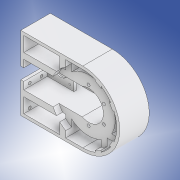
# Autodesk Inventor part: SJ001
Saved by Autodesk Inventor 2017 SP1 (Build 210196100, 196)
## iProperties
Created: 2017-06-03
Part Number: SJ001
Material: ABS Plastic
Document SubType Name: Modeling
Designer: Zach
Density: 1.06 g/cm^3
Appearance: CR White
Author: Zach
Autodesk Inventor part; units mm, degrees
ref_plane "YZ Plane" through (0, 0, 0) normal (1, 0, 0) x (0, 1, 0)
ref_plane "XZ Plane" through (0, 0, 0) normal (0, 1, 0) x (-1, 0, 0)
ref_plane "XY Plane" through (0, 0, 0) normal (0, 0, 1) x (1, 0, 0)
sketch "Sketch1" plane through (0, 0, 0) normal (0, 0, 1) x (1, 0, 0)
  circle A0 centre (0, 0) radius 62.5 construction
  line L0 (0, 62.5) -> (-105, 62.5)
  line L1 (-105, 62.5) -> (-105, -62.5)
  line L2 (-105, -62.5) -> (0, -62.5)
  arc A1 (0, -62.5) -> (0, 62.5) centre (0, 0) ccw
  dimension "d0" = 125
  dimension "d1" = 105
  constraints: 6 end point, 4 point on circle, 4 tangent, 2 centre point, 2 vertical alignment, 1 coincident, 1 concentric, 1 horizontal, 1 perpendicular
  measures "d0" diameter of A0
  measures "d1" distance of L0.start L0.end
extrude "Extrusion1" add sketch "Sketch1" along normal blind 50
sketch "Sketch6" plane through (0, 0, 50) normal (0, 0, 1) x (1, 0, 0)
  circle A0 centre (0, 0) radius 22.5
  arc A1 (0, -62.5) -> (0, 62.5) centre (0, 0) ccw projected
  dimension "d125" = 45
  constraints: 1 centre point, 1 coincident
  measures "d125" diameter of A0
extrude "Extrusion6" cut sketch "Sketch6" against normal blind 40
sketch "Sketch7" plane through (0, 0, 50) normal (0, 0, 1) x (1, 0, 0)
  line L0 (0, 10) -> (-105, 10)
  line L1 (-105, 10) -> (-105, -10)
  line L2 (-105, -10) -> (0, -10)
  line L3 (0, -10) -> (0, 10)
  circle A0 centre (0, 0) radius 22.5 projected
  line L4 (-105, 62.5) -> (-105, -62.5) projected
  point P0 (-105, 0)
  dimension "d28" = 20
  constraints: 8 end point, 3 midpoint, 2 parallel, 1 coincident, 1 horizontal, 1 perpendicular
  measures "d28" distance of L1.end L0.end
extrude "Extrusion7" cut sketch "Sketch7" against normal blind 40 contours L3 L2 A0 L0 | A0 L2 L1 L0 picked at (-7.5, 0)
sketch "Sketch9" plane through (0, 0, 50) normal (0, 0, 1) x (1, 0, 0)
  circle A0 centre (0, 30) radius 2.5
  circle A1 centre (-25.9808, 15) radius 2.5
  circle A2 centre (-25.9808, -15) radius 2.5
  circle A3 centre (0, -30) radius 2.5
  circle A4 centre (25.9808, -15) radius 2.5
  circle A5 centre (25.9808, 15) radius 2.5
  circle A6 centre (0, 0) radius 30 construction
  dimension "d123" = 60
  dimension "d35" = 5
  dimension "d39" = 360
  constraints: 6 centre point, 2 vertical alignment, 1 coincident, 15 other
  measures "d35" diameter of A0
extrude "Extrusion9" cut sketch "Sketch9" against normal through all
sketch "Sketch10" plane through (0, 0, 50) normal (0, 0, 1) x (1, 0, 0)
  circle A0 centre (0, 0) radius 45
  arc A1 (0, -57.5) -> (0, -57.5) centre (0, 0) ccw
  line L0 (0, -57.5) -> (-100, -57.5)
  line L1 (-100, 57.5) -> (-100, -57.5)
  line L2 (0, -57.5) -> (-75, -57.5)
  line L3 (0, 57.5) -> (-100, 57.5)
  circle A2 centre (0, 0) radius 57.5 construction
  arc A3 (0, -57.5) -> (0, 57.5) centre (0, 0) ccw
  line L4 (0, 62.5) -> (-105, 62.5) construction
  line L5 (-105, 62.5) -> (-105, 10) construction
  line L6 (-105, -10) -> (-105, 10) construction
  line L7 (-105, -10) -> (-105, -62.5) construction
  line L8 (-105, -62.5) -> (0, -62.5) construction
  arc A4 (0, -62.5) -> (0, 62.5) centre (0, 0) ccw construction
  point P0 (-100, 0)
  dimension "d111" = 115
  dimension "d43" = 90
  dimension "d114" = 90
  dimension "d124" = 5
  dimension "d212" = 5
  dimension "d213" = 5
  constraints: 8 end point, 4 point on circle, 3 centre point, 3 coincident, 2 tangent, 1 midpoint, 1 perpendicular, 1 vertical alignment, 3 other
  measures "d43" diameter of A0
  measures "d114" angle of L1 L3
  measures "d124" distance between parallel lines of L4 L3
  measures "d212" distance between parallel lines of L8 L0
  measures "d213" distance from line of L6 point (-100, 0)
extrude "Extrusion10" cut sketch "Sketch10" against normal blind 40
sketch "Sketch18" plane through (-105, -62.5, 0) normal (-1, 0, 0) x (0, 0, 1)
  circle A0 centre (40, 45) radius 2.5
  circle A1 centre (20, 45) radius 2.5
  line L0 (0, 125) -> (0, 0)
  circle A2 centre (40, 80) radius 2.5
  circle A3 centre (20, 80) radius 2.5
  circle A4 centre (20, 116.25) radius 2.5
  circle A5 centre (20, 8.75) radius 2.5
  circle A6 centre (40, 8.75) radius 2.5
  circle A7 centre (40, 116.25) radius 2.5
  line L1 (0, 125) -> (50, 125)
  line L2 (10, 87.5) -> (50, 87.5)
  line L3 (10, 52.5) -> (50, 52.5)
  line L4 (0, 0) -> (50, 0)
  line L5 (50, 52.5) -> (50, 37.5)
  point P0 (0, 62.5)
  dimension "d76" = 5
  dimension "d77" = 5
  dimension "d80" = 20
  dimension "d91" = 5
  dimension "d92" = 5
  dimension "d94" = 5
  dimension "d95" = 5
  dimension "d96" = 5
  dimension "d97" = 5
  dimension "d115" = 8.75
  dimension "d116" = 7.5
  dimension "d118" = 8.75
  dimension "d129" = 7.5
  constraints: 12 end point, 8 centre point, 6 vertical alignment, 4 horizontal alignment
  measures "d76" diameter of A0
  measures "d77" diameter of A1
  measures "d80" distance of A1.centre A0.centre
  measures "d91" diameter of A2
  measures "d92" diameter of A3
  measures "d94" diameter of A4
  measures "d95" diameter of A5
  measures "d96" diameter of A6
  measures "d97" diameter of A7
  measures "d115" distance from line of L1 A7.centre
  measures "d116" distance from line of L2 A2.centre
  measures "d118" distance from line of L4 A6.centre
  measures "d129" distance from line of A0.centre L3
extrude "Extrusion39" cut sketch "Sketch18" against normal blind 10
sketch "Sketch46" plane through (0, 0, 10) normal (0, 0, 1) x (1, 0, 0)
  arc A0 (-43.8748, -10) -> (-43.8748, 10) centre (0, 0) ccw construction
  line L0 (-45, 22.5) -> (-100, 22.5)
  line L1 (-31.1247, 32.5) -> (-100, 32.5)
  line L2 (-100, 32.5) -> (-100, 22.5)
  line L3 (-100, 22.5) -> (-31.1247, 22.5)
  line L4 (-31.1247, 22.5) -> (-31.1247, 32.5)
  line L5 (-135.4871, 0) -> (135.4871, 0) construction
  line L6 (-95, 57.5) -> (0, 57.5) construction
  line L7 (-38.9711, 22.5) -> (-28.9711, 22.5)
  line L8 (-28.9711, 22.5) -> (-28.9711, 57.5)
  line L9 (-28.9711, 57.5) -> (-38.9711, 57.5)
  line L10 (-38.9711, 57.5) -> (-38.9711, 22.5)
  arc A1 (0, -57.5) -> (0, 57.5) centre (0, 0) ccw construction
  line L11 (31.1247, 32.5) -> (52.915, 32.5)
  line L12 (52.915, 32.5) -> (52.915, 22.5)
  line L13 (52.915, 22.5) -> (31.1247, 22.5)
  line L14 (31.1247, 22.5) -> (31.1247, 32.5)
  line L15 (31.1247, 22.5) -> (21.1247, 22.5)
  line L16 (21.1247, 22.5) -> (21.1247, 53.4789)
  line L17 (21.1247, 53.4789) -> (31.1247, 53.4789)
  line L18 (31.1247, 53.4789) -> (31.1247, 22.5)
  line L19 (-45, -22.5) -> (-100, -22.5)
  line L20 (-31.1247, -32.5) -> (-100, -32.5)
  line L21 (-100, -32.5) -> (-100, -22.5)
  line L22 (-100, -22.5) -> (-31.1247, -22.5)
  line L23 (-31.1247, -22.5) -> (-31.1247, -32.5)
  line L24 (-28.9711, -22.5) -> (-28.9711, -57.5)
  line L25 (-28.9711, -57.5) -> (-38.9711, -57.5)
  line L26 (-38.9711, -57.5) -> (-38.9711, -22.5)
  line L27 (31.1247, -32.5) -> (52.915, -32.5)
  line L28 (52.915, -32.5) -> (52.915, -22.5)
  line L29 (52.915, -22.5) -> (31.1247, -22.5)
  line L30 (31.1247, -22.5) -> (31.1247, -32.5)
  line L31 (31.1247, -22.5) -> (21.1247, -22.5)
  line L32 (21.1247, -22.5) -> (21.1247, -53.4789)
  line L33 (21.1247, -53.4789) -> (31.1247, -53.4789)
  line L34 (31.1247, -53.4789) -> (31.1247, -22.5)
  line L35 (-28.9711, -22.5) -> (-38.9711, -22.5)
  line L36 (-100, -22.5) -> (5, -22.5) construction
  line L37 (-100, 10) -> (-100, 57.5) construction
  arc A2 (-43.8748, -10) -> (-43.8748, 10) centre (0, 0) ccw projected
  dimension "d229" = 10
  dimension "d230" = 10
  dimension "d231" = 10
  dimension "d232" = 10
  constraints: 74 end point, 15 symmetric about line, 11 point on circle, 8 parallel, 5 horizontal, 4 perpendicular, 3 point on line, 2 centre point, 1 coincident, 1 collinear, 1 horizontal alignment, 1 midpoint
  measures "d229" distance of L1.end L0.end
  measures "d230" distance of L9.end L8.end
  measures "d231" distance of L11.end L12.end
  measures "d232" distance of L16.end L17.end
extrude "Extrusion44" add sketch "Sketch46" along normal blind 40
sketch "Sketch22" plane through (0, 0, 50) normal (0, 0, 1) x (1, 0, 0)
  arc A0 (0, -62.5) -> (0, 62.5) centre (0, 0) ccw projected
  circle A1 centre (0, 0) radius 55
  point P0 (0, 0)
  dimension "d122" = 110
  constraints: 1 centre point, 1 coincident
  measures "d122" diameter of A1
extrude "Extrusion20" cut sketch "Sketch22" against normal blind 10
sketch "Sketch30" plane through (0, 0, 0) normal (0, 0, -1) x (-1, 0, 0)
  circle A0 centre (0, 0) radius 42.5 construction
  line L0 (0, 42.5) -> (105, 42.5)
  line L1 (105, 62.5) -> (105, -62.5) projected
  line L2 (0, -42.5) -> (105, -42.5)
  line L3 (105, 42.5) -> (105, -42.5)
  arc A1 (0, 42.5) -> (0, -42.5) centre (0, 0) ccw
  line L4 (100, 22.5) -> (0, 22.5)
  arc A2 (0, 22.5) -> (0, -22.5) centre (0, 0) ccw
  line L5 (0, -22.5) -> (100, -22.5)
  line L6 (100, -22.5) -> (100, 22.5)
  dimension "d162" = 85
  dimension "d201" = 45
  dimension "d202" = 5
  constraints: 12 end point, 6 point on circle, 3 centre point, 2 parallel, 2 point on line, 2 tangent, 1 coincident, 1 collinear, 1 concentric, 1 horizontal, 2 other
  measures "d162" diameter of A0
  measures "d201" distance between parallel lines of L5 L4
  measures "d202" distance between parallel lines of L1 L6
extrude "Extrusion29" add sketch "Sketch30" along normal blind 5
sketch "Sketch32" plane through (0, 0, 0) normal (0, 0, -1) x (-1, 0, 0)
  arc A0 (0, 22.5) -> (0, -22.5) centre (0, 0) ccw projected
  circle A1 centre (0, 0) radius 22.5 construction
  line L0 (0, 22.5) -> (100, 22.5)
  line L1 (100, -22.5) -> (100, 22.5) projected
  line L2 (0, -22.5) -> (100, -22.5)
  line L3 (100, 22.5) -> (100, -22.5)
  arc A2 (0, 22.5) -> (0, -22.5) centre (0, 0) ccw
  point P0 (0, 0)
  dimension "d168" = 45
  constraints: 6 end point, 4 point on circle, 3 tangent, 2 centre point, 2 horizontal, 2 point on line, 1 coincident, 1 collinear
  measures "d168" diameter of A1
extrude "Extrusion30" cut sketch "Sketch32" against normal through all
sketch "Sketch33" plane through (0, 0, -5) normal (0, 0, -1) x (-1, 0, 0)
  line L0 (100, 22.5) -> (100, -22.5) projected
  line L1 (100, -22.5) -> (0, -22.5) projected
  arc A0 (0, 22.5) -> (0, -22.5) centre (0, 0) ccw projected
  line L2 (0, 22.5) -> (100, 22.5) projected
  arc A1 (0, 42.5) -> (0, -42.5) centre (0, 0) ccw projected
  line L3 (0, -42.5) -> (105, -42.5) projected
  line L4 (105, -42.5) -> (105, 42.5) projected
  line L5 (105, 42.5) -> (0, 42.5) projected
  point P0 (0, 0)
extrude "Extrusion31" add sketch "Sketch33" along normal blind 5 contours L0 L1 A0 L2 | L5 L4 L3 A1
sketch "Sketch37" plane through (0, 0, 10) normal (0, 0, 1) x (1, 0, 0)
  circle A0 centre (0, 0) radius 15
  circle A1 centre (-77.5, 0) radius 12.5
  line L0 (-100, 22.5) -> (-100, -22.5)
  line L1 (-100, -22.5) -> (5, -22.5)
  arc A2 (5, -22.5) -> (5, 22.5) centre (5, 0) ccw
  line L2 (5, 22.5) -> (-100, 22.5)
  line L3 (-93, -15.5) -> (-62, -15.5) construction
  line L4 (-62, -15.5) -> (-62, 15.5) construction
  line L5 (-62, 15.5) -> (-93, 15.5) construction
  line L6 (-93, 15.5) -> (-93, -15.5) construction
  circle A3 centre (-77.5, 0) radius 3 construction
  line L7 (-93, -15.5) -> (-62, 15.5) construction
  line L8 (-62, -15.5) -> (-93, 15.5) construction
  line L9 (-100, -22.5) -> (-55, -22.5)
  line L10 (-55, -22.5) -> (-55, 22.5)
  line L11 (-55, 22.5) -> (-100, 22.5)
  line L12 (-100, 22.5) -> (-100, -22.5)
  line L13 (-100, -22.5) -> (-55, 22.5) construction
  line L14 (-55, -22.5) -> (-100, 22.5) construction
  circle A4 centre (-77.5, 0) radius 3
  circle A5 centre (-62, 15.5) radius 1.5
  circle A6 centre (-93, 15.5) radius 1.5
  circle A7 centre (-93, -15.5) radius 1.5
  circle A8 centre (-62, -15.5) radius 1.5
  point P0 (-77.5, 0)
  dimension "d188" = 31
  dimension "d189" = 45
  dimension "d191" = 31
  dimension "d192" = 6
  dimension "d193" = 3
  dimension "d194" = 3
  dimension "d195" = 3
  dimension "d196" = 3
  dimension "d242" = 25
  constraints: 30 end point, 9 centre point, 8 midpoint, 7 coincident, 4 parallel, 2 horizontal, 2 perpendicular, 2 point on circle
  measures "d188" distance of L5.end L4.end
  measures "d189" distance of L0.start L10.end
  measures "d191" distance of L3.end L4.end
  measures "d192" diameter of A4
  measures "d193" diameter of A5
  measures "d194" diameter of A6
  measures "d195" diameter of A7
  measures "d196" diameter of A8
  measures "d242" diameter of A1
extrude "Extrusion35" add sketch "Sketch37" against normal blind 5 contours L2 L10 L1 L0
sketch "Sketch39" plane through (0, 0, -10) normal (0, 0, -1) x (-1, 0, 0)
  circle A0 centre (77.5, 0) radius 3
  circle A1 centre (77.5, 0) radius 12.5 projected
  circle A2 centre (62, -15.5) radius 1.5 projected
  circle A3 centre (93, -15.5) radius 1.5 projected
  circle A4 centre (93, 15.5) radius 1.5 projected
  circle A5 centre (62, 15.5) radius 1.5 projected
  line L0 (55, -22.5) -> (55, 22.5) construction
  line L1 (100, 22.5) -> (55, 22.5) construction
  circle A6 centre (62, -15.5) radius 1.5 projected
  circle A7 centre (93, -15.5) radius 1.5 projected
  circle A8 centre (93, 15.5) radius 1.5 projected
  circle A9 centre (40.5, 0) radius 4
  circle A10 centre (0, 0) radius 22.5 construction
  circle A11 centre (40.5, 0) radius 22.5 construction
  line L2 (55, -22.5) -> (100, -22.5) projected
  line L3 (105, 10) -> (100, 10) projected
  line L4 (105, -10) -> (105, 10) projected
  line L5 (100, -10) -> (105, -10) projected
  line L6 (100, -22.5) -> (100, -10) projected
  line L7 (100, 10) -> (100, 22.5) projected
  circle A12 centre (0, 0) radius 4
  dimension "d217" = 6
  dimension "d218" = 37
  dimension "d219" = 8
  dimension "d222" = 45
  dimension "d223" = 45
  dimension "d235" = 8
  constraints: 5 centre point, 4 coincident, 1 horizontal alignment
  measures "d217" diameter of A0
  measures "d218" distance of A0.centre A9.centre
  measures "d219" diameter of A9
  measures "d222" diameter of A10
  measures "d223" diameter of A11
  measures "d235" diameter of A12
extrude "Extrusion37" cut sketch "Sketch39" against normal blind 15 contours A0 | A2 | A3 | A4 | A5 | A9 | A12
sketch "Sketch40" plane through (0, 0, 5) normal (0, 0, -1) x (-1, 0, 0)
  circle A0 centre (77.5, 0) radius 12.5 projected
  circle A1 centre (77.5, 0) radius 3
  point P0 (0, 0)
  dimension "d207" = 6
  constraints: 1 centre point, 1 coincident
  measures "d207" diameter of A1
extrude "Extrusion38" add sketch "Sketch40" against normal blind 3
sketch "Sketch44" plane through (0, 0, -10) normal (0, 0, -1) x (-1, 0, 0)
  circle A0 centre (77.5, 0) radius 3 projected
  circle A1 centre (77.5, 0) radius 7.5
  point P0 (0, 0)
  dimension "d224" = 15
  constraints: 1 centre point, 1 coincident
  measures "d224" diameter of A1
extrude "Extrusion42" add sketch "Sketch44" along normal blind 5
sketch "Sketch45" plane through (-77.5, 0, -15) normal (0, 0, -1) x (-1, 0, 0)
  circle A0 centre (0, 0) radius 3 projected
  circle A1 centre (0, 0) radius 7.5 projected
  point P0 (-77.5, 0)
extrude "Extrusion43" add sketch "Sketch45" along normal blind 2 contours A0 | A1
sketch "Sketch47" plane through (-100, 10, 50) normal (1, 0, 0) x (0, 0, -1)
  line L0 (45, 12.5) -> (45, -32.5) projected
  line L1 (60, -2.5) -> (60, -17.5) projected
  line L2 (55, -14) -> (55, -6) projected
  line L3 (55, 4) -> (55, 7) projected
  line L4 (55, -27) -> (55, -24) projected
  line L5 (55, -27) -> (55, -24) projected
  line L6 (55, 4) -> (55, 7) projected
  line L7 (55, -14) -> (55, -6) projected
  line L8 (55, -13) -> (55, -7) projected
  line L9 (55, 12.5) -> (55, -32.5) projected
  line L10 (55, -32.5) -> (55, 12.5) projected
  line L11 (45, -32.5) -> (55, -32.5)
  line L12 (55, -32.5) -> (55, 12.5)
  line L13 (55, 12.5) -> (45, 12.5)
  line L14 (45, 12.5) -> (45, -32.5)
  line L15 (40, -32.5) -> (40, -20) projected
  line L16 (0, -20) -> (40, -20) projected
  line L17 (0, -32.5) -> (0, -20) projected
  line L18 (0, -32.5) -> (40, -32.5) projected
  circle A0 centre (10, -27.5) radius 2.5 projected
  circle A1 centre (30, -27.5) radius 2.5 projected
  line L19 (40, 0) -> (0, 0) projected
  line L20 (40, 0) -> (40, 12.5) projected
  line L21 (40, 12.5) -> (0, 12.5) projected
  line L22 (0, 0) -> (0, 12.5) projected
  line L23 (40, 0) -> (0, 0) projected
  circle A2 centre (30, 7.5) radius 2.5 projected
  circle A3 centre (10, 7.5) radius 2.5 projected
  point P0 (50, -10)
  constraints: 8 end point, 2 horizontal alignment, 2 parallel, 2 point on line, 1 horizontal, 1 perpendicular
extrude "Extrusion45" cut sketch "Sketch47" against normal through all contours L13 L9 L3 L2 L4 L11 L0
sketch "Sketch42" plane through (0, 0, -10) normal (0, 0, -1) x (-1, 0, 0)
  circle A0 centre (40.5, 0) radius 4 projected
  circle A1 centre (93, 15.5) radius 1.5 projected
  circle A2 centre (62, -15.5) radius 1.5 projected
  circle A3 centre (93, -15.5) radius 1.5 projected
  circle A4 centre (62, 15.5) radius 1.5 projected
  arc A5 (0, 42.5) -> (0, -42.5) centre (0, 0) ccw projected
  line L0 (0, -42.5) -> (105, -42.5) projected
  line L1 (105, -42.5) -> (105, 42.5) projected
  line L2 (105, 42.5) -> (0, 42.5) projected
  point P0 (0, 0)
extrude "Extrusion41" [suppressed]
sketch "Sketch48" plane through (0, 0, 50) normal (0, 0, 1) x (1, 0, 0)
  arc A0 (0, -22.5) -> (0, 22.5) centre (0, 0) ccw
  circle A1 centre (0, 0) radius 25
  circle A2 centre (-40.5, 0) radius 4
  circle A3 centre (-40.5, 0) radius 25
  dimension "d238" = 50
  dimension "d241" = 50
  constraints: 4 centre point, 2 coincident, 2 point on circle
  measures "d238" diameter of A1
  measures "d241" diameter of A3
extrude "Extrusion46" cut sketch "Sketch48" against normal blind 55 contours A1 A3 | A3 A1 | A2 picked at (11.2831, -1.8887) picked at (-18.8478, 1.728)
body "Solid1"
